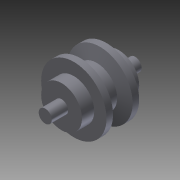
# Autodesk Inventor part: 3464
Saved by Autodesk Inventor 2011 SP1 (Build 150282100, 282)
## iProperties
Created: 2011-09-28
Part Number: 3464
Cost Center: 0 kg
Material: Steel
Document SubType Name: Modeling
Designer: PMe
Authority: 0 mm^3
Stock Number: =<Filenr>_<Document number>
Density: 7.85 g/cm^3
Company: Allseas Engineering BV
Subject: =<Title><TITLE 1_2> <TITLE 2_2>
Author: PMe
Act. Code: DW000
SaveDate: 2011-07-28
SaveTime: 18:32
FileName: Standard
TotalMass: 0 kg
TotalVolume: 0 mm^3
Autodesk Inventor part; units mm, degrees
ref_plane "YZ Plane" through (0, 0, 0) normal (1, 0, 0) x (0, 1, 0)
ref_plane "XZ Plane" through (0, 0, 0) normal (0, 1, 0) x (-1, 0, 0)
ref_plane "XY Plane" through (0, 0, 0) normal (0, 0, 1) x (1, 0, 0)
sketch "Sketch1" plane through (0, 0, 0) normal (0, 0, 1) x (1, 0, 0)
  line L0 (0, -5.5) -> (0, 5.5)
  line L1 (0, 5.5) -> (-0.8, 5.5)
  line L2 (-0.8, 5.5) -> (-0.8, 3.5)
  line L3 (-0.8, 3.5) -> (-2.5, 3.5)
  line L4 (-2.5, 3.5) -> (-2.5, 2)
  line L5 (-2.5, 2) -> (-4, 2)
  line L6 (-4, 2) -> (-4, 1.2)
  line L7 (-4, 1.2) -> (-2.5, 0.8)
  line L8 (-2.5, 0.8) -> (-2.5, -0.8)
  line L9 (-2.5, -0.8) -> (-4, -1.2)
  line L10 (-4, -1.2) -> (-4, -2)
  line L11 (-4, -2) -> (-2.5, -2)
  line L12 (-2.5, -2) -> (-2.5, -3.5)
  line L13 (-2.5, -3.5) -> (-0.8, -3.5)
  line L14 (-0.8, -3.5) -> (-0.8, -5.5)
  line L15 (-0.8, -5.5) -> (0, -5.5)
  point P0 (0, 0)
  point P1 (0, 0)
  point P2 (-2.5, 0)
  dimension "d0" = 11
  dimension "d1" = 5
  dimension "d2" = 1.6
  dimension "d3" = 7
  dimension "d4" = 8
  dimension "d5" = 4
  dimension "d6" = 1.6
  dimension "d7" = 0.8
  constraints: 32 end point, 6 parallel, 6 perpendicular, 4 equal length, 4 vertical alignment, 2 midpoint, 1 coincident, 1 collinear, 1 horizontal alignment, 1 vertical
  measures "d0" distance of L0.start L0.end
  measures "d1" diameter of L12 L0
  measures "d2" diameter of L14 L0
  measures "d3" distance between parallel lines of L3 L13
  measures "d4" diameter of L6 L0
  measures "d5" distance between parallel lines of L11 L5
  measures "d6" distance of L7.end L8.end
  measures "d7" distance of L9.end L10.end
revolve "Revolution1" add sketch "Sketch1" angle 360 about axis through (0, -5.5, 0) along (0, 1, 0)
body "Solid1"
